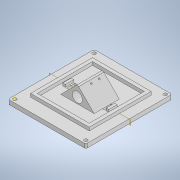
# Autodesk Inventor part: Senzor-vikos
Saved by Autodesk Inventor 2022 (Build 260153000, 153)
## iProperties
Created: 2023-05-16
Part Number: Senzor-vikos
Material: Všeobecné
Document SubType Name: Modeling
Designer: Tada
Density: 1 g/cm^3
Appearance: Výchozí
Author: Tada
Autodesk Inventor part; units mm, degrees
ref_plane "YZ Plane" through (0, 0, 0) normal (1, 0, 0) x (0, 1, 0)
ref_plane "XZ Plane" through (0, 0, 0) normal (0, 1, 0) x (-1, 0, 0)
ref_plane "XY Plane" through (0, 0, 0) normal (0, 0, 1) x (1, 0, 0)
sketch "Náčrt1" plane through (0, 0, 0) normal (0, 1, 0) x (-1, 0, 0)
  line L0 (0, 0) -> (-85, 0)
  line L1 (-85, 0) -> (-85, -95)
  line L2 (-85, -95) -> (0, -95)
  line L3 (0, -95) -> (0, 0)
  line L4 (4, 4) -> (-89, 4)
  line L5 (-89, 4) -> (-89, -99)
  line L6 (-89, -99) -> (4, -99)
  line L7 (4, -99) -> (4, 4)
  circle A0 centre (0, 0) radius 2
  circle A1 centre (0, -95) radius 2
  circle A2 centre (-85, -95) radius 2
  circle A3 centre (-85, 0) radius 2
  dimension "d0" = 4
  dimension "d1" = 4
  dimension "d2" = 4
  dimension "d3" = 4
  dimension "d4" = 85
  dimension "d5" = 95
  dimension "d6" = 4
  dimension "d7" = 4
  dimension "d8" = 4
  dimension "d9" = 4
  dimension "d10" = 4
  dimension "d11" = 4
  constraints: 16 end point, 4 centre point, 4 parallel, 3 coincident, 2 horizontal, 2 perpendicular
  measures "d0" distance between parallel lines of L7 L3
  measures "d1" distance between parallel lines of L6 L2
  measures "d2" distance between parallel lines of L1 L5
  measures "d3" distance between parallel lines of L4 L0
  measures "d4" distance of L1.end L2.end
  measures "d5" distance of L0.end L1.end
  measures "d6" diameter of A0
  measures "d7" distance from line of L4 A0.centre
  measures "d8" distance from line of L7 A0.centre
  measures "d9" diameter of A1
  measures "d10" diameter of A2
  measures "d11" diameter of A3
extrude "Vysunutí1" add sketch "Náčrt1" along normal blind 5 contours L0 A0 L3 A1 L2 A2 L1 A3 | L7 L6 L5 L4
extrude "Vysunutí2" cut sketch "Náčrt1" along normal blind 5 contours A3 L1 L0 | L0 L1 A3 | A0 L3 L0 | L0 L3 A0 | A2 L2 L1 | L1 L2 A2 | A1 L2 L3 | L3 L2 A1
fillet "Zaoblení1" radius 2 4 edges at (89, 2.5, 4) (-4, 2.5, 4) (89, 2.5, -99) (-4, 2.5, -99)
sketch "Náčrt2" plane through (0, 5, 0) normal (0, 1, 0) x (1, 0, 0)
  point P0 (0, 0)
ref_plane "Pracovní rovina1" through (87, 0, -47.5) normal (0, 0, -1) x (-1, 0, 0)
sketch "Náčrt3" plane through (87, 0, -47.5) normal (0, 0, -1) x (-1, 0, 0)
  line L0 (89, 5) -> (0, 5) projected
  line L1 (24.5, 5) -> (64.5, 5)
  line L2 (64.5, 5) -> (44.5, 25)
  line L3 (44.5, 25) -> (24.5, 5)
  line L4 (24.5, 5) -> (64.5, 5)
  line L5 (91, 0) -> (91, 5) projected
  point P0 (87, 0)
  dimension "d22" = 90
  dimension "d26" = 45
  dimension "d27" = 20
  dimension "d28" = 46.5
  constraints: 8 end point, 2 point on line, 1 collinear
  measures "d22" angle of L3 L2
  measures "d26" angle of L2 L0
  measures "d27" distance from line of L0 L2.end
  measures "d28" distance from line of L5 L2.end
extrude "Vysunutí3" add sketch "Náčrt3" along normal mid plane 30
fillet "Zaoblení2" radius 2 1 edges at (42.5, 25, -47.5)
sketch "Náčrt4" plane through (0, 5, 0) normal (0, 1, 0) x (1, 0, 0)
  line L0 (11.5, 15.5) -> (73.5, 15.5)
  line L1 (73.5, 15.5) -> (73.5, 81.5)
  line L2 (73.5, 81.5) -> (11.5, 81.5)
  line L3 (11.5, 81.5) -> (11.5, 15.5)
  line L4 (7.5, 11.5) -> (77.5, 11.5)
  line L5 (77.5, 11.5) -> (77.5, 85.5)
  line L6 (77.5, 85.5) -> (7.5, 85.5)
  line L7 (7.5, 85.5) -> (7.5, 11.5)
  line L8 (-22.6, 47.5) -> (107.6, 47.5) projected
  line L9 (-4, 97) -> (-4, -2) projected
  line L10 (89, -2) -> (89, 97) projected
  point P0 (0, 0)
  dimension "d32" = 62
  dimension "d33" = 66
  dimension "d34" = 4
  dimension "d35" = 4
  dimension "d36" = 4
  dimension "d37" = 4
  dimension "d38" = 34
  dimension "d39" = 11.5
  dimension "d40" = 11.5
  constraints: 16 end point, 4 parallel, 2 horizontal, 2 perpendicular
  measures "d32" distance of L1.end L2.end
  measures "d33" distance of L0.end L1.end
  measures "d34" distance between parallel lines of L6 L2
  measures "d35" distance between parallel lines of L7 L3
  measures "d36" distance between parallel lines of L4 L0
  measures "d37" distance between parallel lines of L1 L5
  measures "d38" distance between parallel lines of L8 L2
  measures "d39" distance between parallel lines of L9 L7
  measures "d40" distance between parallel lines of L5 L10
extrude "Vysunutí4" add sketch "Náčrt4" along normal blind 4 contours L0 L1 L8 L5 L4 L7 L3 | L8 L7 L6 L5 L1 L2 L3
sketch "Náčrt5" plane through (0, 5, 0) normal (0, 1, 0) x (1, 0, 0)
  line L0 (67, 42.5) -> (70, 42.5)
  line L1 (70, 42.5) -> (70, 52.5)
  line L2 (70, 52.5) -> (67, 52.5)
  line L3 (67, 52.5) -> (67, 42.5)
  line L4 (73.5, 81.5) -> (73.5, 15.5) projected
  line L5 (-22.6, 47.5) -> (107.6, 47.5) projected
  line L6 (15, 42.5) -> (18, 42.5)
  line L7 (18, 42.5) -> (18, 52.5)
  line L8 (18, 52.5) -> (15, 52.5)
  line L9 (15, 52.5) -> (15, 42.5)
  line L10 (11.5, 15.5) -> (11.5, 81.5) projected
  point P0 (0, 0)
  dimension "d43" = 3.5
  dimension "d44" = 3
  dimension "d45" = 10
  dimension "d46" = 5
  dimension "d47" = 5
  dimension "d48" = 10
  dimension "d49" = 3
  dimension "d50" = 3.5
  constraints: 16 end point, 4 parallel, 2 horizontal, 2 perpendicular
  measures "d43" distance between parallel lines of L1 L4
  measures "d44" distance between parallel lines of L3 L1
  measures "d45" distance between parallel lines of L0 L2
  measures "d46" distance between parallel lines of L5 L2
  measures "d47" distance between parallel lines of L8 L5
  measures "d48" distance between parallel lines of L6 L8
  measures "d49" distance between parallel lines of L9 L7
  measures "d50" distance between parallel lines of L10 L9
extrude "Vysunutí5" add sketch "Náčrt5" along normal blind 3
sketch "Náčrt6" plane through (62.5, 5, -62.5) normal (0.7071, 0.7071, 0) x (-0.7071, 0.7071, 0)
  circle A0 centre (23.2843, 17) radius 1
  circle A1 centre (23.2843, 7.5) radius 1
  line L0 (26.2843, 0) -> (0, 0) projected
  line L1 (26.2843, 30) -> (26.2843, 0) projected
  point P0 (40.6586, 62.5)
  dimension "d53" = 9.5
  dimension "d54" = 2
  dimension "d55" = 2
  dimension "d56" = 7.5
  dimension "d57" = 3
  dimension "d58" = 3
  constraints: 2 centre point
  measures "d53" distance of A0.centre A1.centre
  measures "d54" diameter of A1
  measures "d55" diameter of A0
  measures "d56" distance from line of L0 A1.centre
  measures "d57" distance from line of L1 A0.centre
  measures "d58" distance from line of L1 A1.centre
sketch "Náčrt7" plane through (22.5, 5, -62.5) normal (-0.7071, 0.7071, 0) x (-0.7071, -0.7071, 0)
  circle A0 centre (-23.2843, 13) radius 1
  circle A1 centre (-23.2843, 22.5) radius 1
  line L0 (-26.2843, 0) -> (-26.2843, 30) projected
  line L1 (-26.2843, 30) -> (0, 30) projected
  point P0 (19.4454, 62.5)
  dimension "d59" = 2
  dimension "d60" = 2
  dimension "d61" = 9.5
  dimension "d62" = 3
  dimension "d63" = 3
  dimension "d64" = 7.5
  constraints: 2 centre point
  measures "d59" diameter of A1
  measures "d60" diameter of A0
  measures "d61" distance of A0.centre A1.centre
  measures "d62" distance from line of L0 A1.centre
  measures "d63" distance from line of L0 A0.centre
  measures "d64" distance from line of L1 A1.centre
extrude "Vysunutí6" cut sketch "Náčrt6" against normal blind 5
extrude "Vysunutí7" cut sketch "Náčrt7" against normal blind 5
sketch "Náčrt8" plane through (0, 5, 0) normal (0, 1, 0) x (1, 0, 0)
  line L0 (62.5, 62.5) -> (62.5, 32.5) projected
  line L1 (62.5, 42.5) -> (65.5, 42.5)
  line L2 (65.5, 42.5) -> (65.5, 52.5)
  line L3 (65.5, 52.5) -> (62.5, 52.5)
  line L4 (62.5, 52.5) -> (62.5, 42.5)
  line L5 (70, 52.5) -> (67, 52.5) projected
  line L6 (67, 42.5) -> (70, 42.5) projected
  line L7 (-22.6, 47.5) -> (107.6, 47.5) projected
  line L8 (22.5, 32.5) -> (22.5, 62.5) projected
  line L9 (22.5, 42.5) -> (19.5, 42.5)
  line L10 (19.5, 42.5) -> (19.5, 52.5)
  line L11 (19.5, 52.5) -> (22.5, 52.5)
  line L12 (22.5, 52.5) -> (22.5, 42.5)
  line L13 (15, 42.5) -> (18, 42.5) projected
  point P0 (0, 0)
  dimension "d69" = 10
  dimension "d70" = 5
  dimension "d73" = 5
  dimension "d74" = 10
  constraints: 16 end point, 4 parallel, 3 collinear, 2 horizontal, 2 perpendicular, 2 point on line
  measures "d69" distance between parallel lines of L1 L3
  measures "d70" distance between parallel lines of L3 L7
  measures "d73" distance between parallel lines of L9 L7
  measures "d74" distance between parallel lines of L11 L9
extrude "Vysunutí8" cut sketch "Náčrt8" against normal blind 5 contours L3 L2 L7 L0 | L7 L2 L1 L0
extrude "Vysunutí9" cut sketch "Náčrt8" against normal blind 5 contours L8 L9 L10 L7 | L7 L10 L11 L8
sketch "Náčrt9" plane through (87, 0, -62.5) normal (0, 0, -1) x (-1, 0, 0)
  circle A0 centre (44.6005, 12.1716) radius 6
  arc A1 (45.9142, 23.5858) -> (43.0858, 23.5858) centre (44.5, 22.1716) ccw projected
  line L0 (64.5, 5) -> (45.9142, 23.5858) projected
  line L1 (43.0858, 23.5858) -> (24.5, 5) projected
  point P0 (87, 0)
  dimension "d77" = 12
  dimension "d78" = 10
  dimension "d79" = 9
  dimension "d80" = 9.1421
  constraints: 1 centre point
  measures "d77" diameter of A0
  measures "d78" vertical distance of A1.centre A0.centre
  measures "d79" distance from line of L0 A0.centre
  measures "d80" distance from line of L1 A0.centre
extrude "Vysunutí10" cut sketch "Náčrt9" against normal blind 30
equation "\"d1\" = d0"
equation "\"d2\" = d0"
equation "\"d3\" = d0"
equation "\"d9\" = d7"
equation "\"d10\" = d7"
equation "\"d11\" = d7"
equation "\"d35\" = d34"
equation "\"d36\" = d34"
equation "\"d37\" = d34"
equation "\"d55\" = d54"
equation "\"d58\" = d57"
equation "\"d60\" = d59"
equation "\"d63\" = d62"
